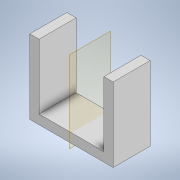
# Autodesk Inventor part: forkV01
Saved by Autodesk Inventor 2020.3 (Build 243373000, 373)
## iProperties
Created: 2020-05-23
Part Number: forkV01
Material: Generic
Document SubType Name: Modeling
Designer: robst
Density: 1 g/cm^3
Appearance: Default
Author: robst
Autodesk Inventor part; units mm, degrees
ref_plane "XZ Plane" through (0, 0, 0) normal (0, 1, 0) x (-1, 0, 0)
ref_plane "XY Plane" through (0, 0, 0) normal (0, 0, 1) x (1, 0, 0)
sketch "Sketch3" plane through (0, 0, 0) normal (0, 0, 1) x (1, 0, 0)
  line L0 (0, 0) -> (0, 127) construction
  line L1 (0, 0) -> (114.3, 0)
  line L2 (114.3, 0) -> (114.3, 203.2)
  line L3 (114.3, 203.2) -> (88.9, 203.2)
  line L4 (88.9, 203.2) -> (88.9, 25.4)
  line L5 (88.9, 25.4) -> (0, 25.4)
  line L6 (0, 25.4) -> (0, 0)
  dimension "d2" = 127
  dimension "armMaterialWidth" = 25.4
  dimension "oneHalfTubeDiameter" = 88.9
  dimension "baseMaterialWidth" = 25.4
  dimension "d6" = 203.2
  constraints: 14 end point, 4 perpendicular, 1 collinear, 1 horizontal, 1 point on line, 1 vertical
  measures "d2" distance of L0.start L0.end
  measures "armMaterialWidth" distance between parallel lines of L4 L2
  measures "oneHalfTubeDiameter" distance between parallel lines of L4 L0
  measures "baseMaterialWidth" distance between parallel lines of L5 L1
  measures "d6" distance between parallel lines of L3 L1
extrude "Extrusion1" add sketch "Sketch3" along normal mid plane 101.6
mirror "Mirror1" about plane through (0, 0, 0) normal (1, 0, 0) of "Extrusion1"
body "Solid1"
